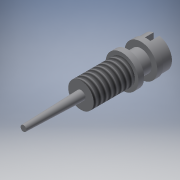
# Autodesk Inventor part: Fuel Intake Adjuster Pin
Saved by Autodesk Inventor 2019 Beta2 (Build 230110000, 110) ContinuousBuild 0
## iProperties
Created: 2012-08-14
Part Number: Fuel Intake Adjuster Pin
Material: Generic
Document SubType Name: Modeling
Designer: John
Density: 1 g/cm^3
Appearance: Default
Author: John
Autodesk Inventor part; units mm, degrees
ref_plane "YZ Plane" through (0, 0, 0) normal (1, 0, 0) x (0, 1, 0)
ref_plane "XZ Plane" through (0, 0, 0) normal (0, 1, 0) x (-1, 0, 0)
ref_plane "XY Plane" through (0, 0, 0) normal (0, 0, 1) x (1, 0, 0)
sketch "Sketch1" plane through (0, 0, 0) normal (1, 0, 0) x (0, 1, 0)
  line L0 (0, 0) -> (0, -2.5116) construction
  line L1 (0, 0) -> (2.3876, 0)
  line L2 (2.3876, 0) -> (2.3876, 1.524)
  line L3 (2.3876, 1.524) -> (2.54, 1.524)
  line L4 (2.54, 1.524) -> (2.54, 2.413)
  line L5 (2.54, 2.413) -> (1.651, 2.413)
  line L6 (1.651, 2.413) -> (1.651, 4.445)
  line L7 (1.651, 4.445) -> (2.54, 4.445)
  line L8 (2.54, 4.445) -> (2.54, 5.334)
  line L9 (2.54, 5.334) -> (1.9685, 5.334)
  line L10 (1.9685, 5.334) -> (1.9685, 11.684)
  line L11 (1.9685, 11.684) -> (0.6985, 11.684)
  line L12 (0.6985, 11.684) -> (0.4445, 20.574)
  line L13 (0.4445, 20.574) -> (0, 20.574)
  line L14 (0, 20.574) -> (0, 0)
  dimension "d0" = 4.7752
  dimension "d2" = 5.08
  dimension "d3" = 3.302
  dimension "d4" = 3.937
  dimension "d5" = 1.397
  dimension "d6" = 0.889
  dimension "d7" = 1.524
  dimension "d8" = 2.413
  dimension "d9" = 4.445
  dimension "d10" = 5.334
  dimension "d11" = 11.684
  dimension "d12" = 20.574
  constraints: 30 end point, 11 parallel, 2 perpendicular, 1 collinear, 1 vertical
  measures "d0" diameter of L2 L0
  measures "d2" diameter of L4 L0
  measures "d3" diameter of L6 L0
  measures "d4" diameter of L10 L0
  measures "d5" diameter of L11.end L0
  measures "d6" diameter of L12.end L0
  measures "d7" distance between parallel lines of L3 L1
  measures "d8" distance between parallel lines of L1 L5
  measures "d9" distance between parallel lines of L1 L7
  measures "d10" distance between parallel lines of L1 L9
  measures "d11" distance between parallel lines of L1 L11
  measures "d12" distance between parallel lines of L1 L13
revolve "Revolution1" add sketch "Sketch1" angle 360 about axis through (0, 0, 0) along (0, 0, -1)
sketch "Sketch2" plane through (0, 0, 0) normal (0, 0, -1) x (-1, 0, 0)
  circle A0 centre (0, 0) radius 2.3876 projected
  line L0 (-0.4445, 2.3876) -> (0.4445, 2.3876)
  line L1 (0.4445, 2.3876) -> (0.4445, -2.3876)
  line L2 (0.4445, -2.3876) -> (-0.4445, -2.3876)
  line L3 (-0.4445, -2.3876) -> (-0.4445, 2.3876)
  dimension "d14" = 0.889
  dimension "d16" = 0.4445
  constraints: 8 end point, 2 parallel, 2 tangent, 1 horizontal, 1 perpendicular
  measures "d14" distance of L0.start L0.end
  measures "d16" distance from line of L1 A0.centre
extrude "Extrusion1" cut sketch "Sketch2" against normal blind 1.524 contours L1 A0 L3 | A0 L0 L1 | L1 L2 A0 | A0 L3 L0 | L2 L3 A0
thread "Thread1" size "8-32 UNC" class "2A" standard "ANSI Unified Screw Threads" full length
equation "\"d16\" = 0.5 * d14"
body "Solid1"
